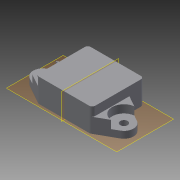
# Autodesk Inventor part: TPS
Saved by Autodesk Inventor 2015 (Build 190159000, 159)
## iProperties
Created: 2015-07-10
Part Number: TPS
Material: Generic
Description: insert part description/title
Document SubType Name: Modeling
Designer: francis
Density: 1 g/cm^3
Appearance: Default
Author: francis
Part Category: insert part category here and press enter to fill value
Autodesk Inventor part; units mm, degrees
ref_plane "XZ Plane" through (0, 0, 0) normal (0, 1, 0) x (-1, 0, 0)
sketch "Sketch1" plane through (0, 0, 0) normal (0, 0, 1) x (1, 0, 0)
  line L0 (-19, 16.7257) -> (19, 16.7257)
  line L1 (19, 16.7257) -> (19, -18.2743)
  line L2 (19, -18.2743) -> (-19, -18.2743)
  line L3 (-19, -18.2743) -> (-19, 16.7257)
  line L4 (0, 21.1891) -> (0, -25.1053) construction
  line L5 (31.0331, 0) -> (-23.8841, 0) construction
  point P0 (0, 0)
  dimension "d0" = 38
  dimension "d1" = 35
  constraints: 12 end point, 2 horizontal, 2 parallel, 1 perpendicular, 1 vertical, 1 other
  measures "d0" distance of L1.end L2.end
  measures "d1" distance of L0.end L1.end
extrude "Extrusion1" add sketch "Sketch1" along normal blind 16
fillet "Fillet1" radius 2 4 edges at (19, 16.7257, 8) (19, -18.2743, 8) (-19, 16.7257, 8) (-19, -18.2743, 8)
sketch "Sketch2" plane through (0, 0, 0) normal (0, 0, 1) x (1, 0, 0)
  line L0 (-19, 14.7257) -> (-19, -16.2743) projected
  line L1 (17, 16.7257) -> (-17, 16.7257) projected
  line L2 (19, -16.2743) -> (19, 14.7257) projected
  line L3 (-17, -18.2743) -> (17, -18.2743) projected
  arc A0 (30.6631, -10.9527) -> (30.6631, 0.4041) centre (27.5, -5.2743) ccw
  line L4 (30.6631, 0.4041) -> (19, 6.901)
  line L5 (-28.9465, 0) -> (40.6791, 0) projected
  line L6 (0, 23.9357) -> (0, -26.5345) projected
  arc A1 (17, -18.2743) -> (19, -16.2743) centre (17, -16.2743) ccw projected
  line L7 (30.6631, -10.9527) -> (17.9733, -18.0215)
  line L8 (19, 6.901) -> (19, -16.2743)
  arc A2 (17.9733, -18.0215) -> (19, -16.2743) centre (17, -16.2743) ccw
  point P0 (0, 0)
  dimension "d5" = 27.5
  dimension "d6" = 13
  dimension "d7" = 6.5
  dimension "d8" = 29.12
  dimension "d9" = 29.12
  constraints: 6 end point, 6 point on circle, 3 tangent, 2 centre point, 1 concentric, 1 point on line, 1 vertical
  measures "d5" distance from line of A0.centre L6
  measures "d6" distance from line of L3 A0.centre
  measures "d7" radius of A0
  measures "d8" angle of L7 L5
  measures "d9" angle of L5 L4
extrude "Extrusion2" add sketch "Sketch2" along normal blind 10 contours L2 L5 A0 L7 A1 | L2 L4 A0 L5
sketch "Sketch3" plane through (0, 0, 10) normal (0, 0, 1) x (1, 0, 0)
  arc A0 (30.6631, -10.9527) -> (30.6631, 0.4041) centre (27.5, -5.2743) ccw construction
  point P0 (0, 0)
  constraints: 1 coincident
hole "Hole1" at (27.5, -5.2743, 10) direction (0, 0, -1) diameter 16 depth 5.4
mirror "Mirror1" about plane through (0, 0, 0) normal (1, 0, 0) of "Extrusion2", "Hole1"
sketch "Sketch4" plane through (27.5, -5.2743, 4.6) normal (0, 0, 1) x (1, 0, 0)
  arc A0 (3.1631, -5.6784) -> (3.1631, 5.6784) centre (0, 0) ccw construction
  line L0 (-58.1631, 5.6784) -> (-54.0889, 7.9479) construction
  arc A1 (-58.1631, 5.6784) -> (-58.1631, -5.6784) centre (-55, 0) ccw construction
  line L1 (-54.0889, -7.9479) -> (-58.1631, -5.6784) construction
  arc A2 (-54.0889, -7.9479) -> (-54.0889, 7.9479) centre (-55, 0) ccw construction
  point P0 (-27.5, 5.2743)
hole "Hole2" at (27.5, -5.2743, 4.6) direction (0, 0, -1) diameter 5 end through all
sketch "Sketch5" plane through (-27.5, -5.2743, 4.6) normal (0, 0, 1) x (1, 0, 0)
  arc A0 (-3.1631, 5.6784) -> (-3.1631, -5.6784) centre (0, 0) ccw construction
  point P0 (27.5, 5.2743)
hole "Hole3" at (-27.5, -5.2743, 4.6) direction (0, 0, -1) diameter 4.5 end through all
equation "\"d9\" = d8"
body "Solid1"
